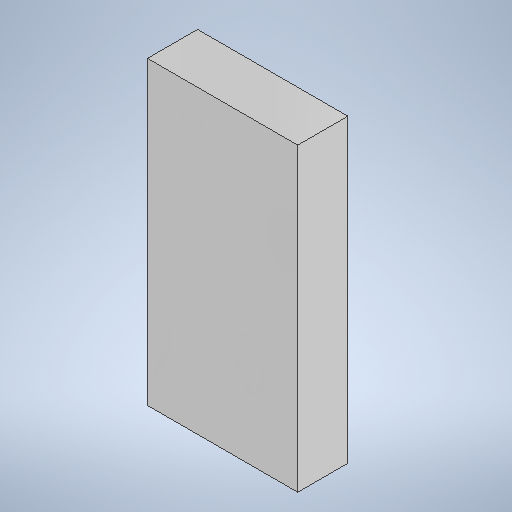
# Autodesk Inventor part: MoldeDerechoPiezaInferiorBarco
Saved by Autodesk Inventor 2025.2 (Build 292293000, 293)
## iProperties
Created: 2025-01-18
Part Number: MoldeDerechoPiezaInferiorBarco
Material: Genérico
Document SubType Name: Modeling
Designer: usuario
Density: 1 g/cm^3
Appearance: Aluminio - Pulido
Author: usuario
Autodesk Inventor part; units mm, degrees
ref_plane "YZ Plane" through (0, 0, 0) normal (1, 0, 0) x (0, 1, 0)
ref_plane "XZ Plane" through (0, 0, 0) normal (0, 1, 0) x (-1, 0, 0)
ref_plane "XY Plane" through (0, 0, 0) normal (0, 0, 1) x (1, 0, 0)
sketch "Boceto1" plane through (0, 0, 0) normal (0, 0, 1) x (1, 0, 0)
  line L0 (0, 0) -> (90, 0)
  line L1 (90, 0) -> (90, 180)
  line L2 (90, 180) -> (0, 180)
  line L3 (0, 180) -> (0, 0)
  line L4 (27.082, 144.48) -> (62.918, 144.48)
  line L5 (62.918, 144.48) -> (62.918, 122.39)
  line L6 (62.918, 122.39) -> (27.082, 122.39)
  line L7 (27.082, 122.39) -> (27.082, 144.48)
  point P0 (45, 144.48)
  dimension "d0" = 180
  dimension "d1" = 90
  dimension "d2" = 35.52
  dimension "d3" = 22.09
  dimension "d4" = 35.836
  dimension "d5" = 45
  constraints: 16 end point, 4 parallel, 2 horizontal, 2 perpendicular, 1 midpoint
  measures "d0" distance of L0.end L1.end
  measures "d1" distance of L0.start L0.end
  measures "d2" distance between parallel lines of L2 L4
  measures "d3" distance of L4.end L5.end
  measures "d4" distance of L5.end L6.end
  measures "d5" distance from line of L3 point (45, 144.48)
sketch "Boceto2" plane through (0, 0, 0) normal (0, 0, 1) x (1, 0, 0)
  line L0 (0, 0) -> (90, 0)
  line L1 (90, 0) -> (90, 180)
  line L2 (90, 180) -> (0, 180)
  line L3 (0, 180) -> (0, 0)
  dimension "d6" = 90
  dimension "d7" = 180
  constraints: 8 end point, 2 parallel, 1 horizontal, 1 perpendicular
  measures "d6" distance of L1.end L2.end
  measures "d7" distance of L0.end L1.end
extrude "Extrusión1" add sketch "Boceto2" along normal blind 30
extrude "Extrusión2" add sketch "Boceto1" against normal blind 10 contours L4 L5 L6 L7
